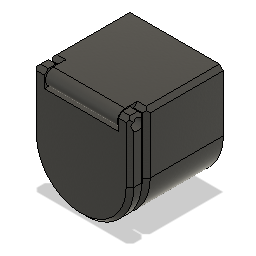
pipowerbuttoncover v2 (Autodesk Fusion 360 design; units mm, degrees)
Autodesk Fusion 360 part; units mm, degrees
sketch "Sketch1" plane through (0, 0, 0) normal (0, 0, 1) x (1, 0, 0)
  circle A0 centre (0, 0) radius 6.1
  circle A1 centre (0, 0) radius 12.5
  line L0 (-12.5, 0) -> (12.5, 0)
  line L1 (12.5, 0) -> (12.5, 12.5)
  line L2 (12.5, 12.5) -> (-12.5, 12.5)
  line L3 (-12.5, 12.5) -> (-12.5, 0)
  dimension "d1" = 12.2
  dimension "d2" = 25
  constraint coincident A0.centre A1.centre
  constraint horizontal L0
  constraint vertical L1
  constraint horizontal L2
  constraint vertical L3
  constraint midpoint A0.centre L0
  constraint coincident A1 L0.start
  constraint tangent A1 L2
  measures "d1" diameter of A0
  measures "d2" diameter of A1
extrude "Extrude1" add sketch "Sketch1" along normal blind 1 contours A0 A1 L0 | A0 A1 L0 | A1 L1 L2 | A1 L2 L3 makes body 1
sketch "Sketch2" plane through (0, 0, 1) normal (0, 0, 1) x (1, 0, 0)
  circle A0 centre (0, 0) radius 6.1
  line L0 (-12.5, 12.5) -> (-12.5, 0)
  arc A1 (-12.5, 0) -> (12.5, 0) centre (0, 0) ccw
  line L1 (12.5, 0) -> (12.5, 12.5)
  line L2 (12.5, 12.5) -> (-12.5, 12.5)
  circle A2 centre (0, 0) radius 10
  line L3 (-10, 0) -> (10, 0)
  line L4 (10, 0) -> (10, 10)
  line L5 (10, 10) -> (-10, 10)
  line L6 (-10, 10) -> (-10, 0)
  dimension "d5" = 20
  constraint concentric A0 A2
  constraint horizontal L3
  constraint vertical L4
  constraint horizontal L5
  constraint vertical L6
  constraint coincident A2 L3.start
  constraint midpoint A0.centre L3
  constraint tangent A2 L5
  measures "d5" diameter of A2
extrude "Extrude2" add sketch "Sketch2" along normal blind 19 bodies 1
extrude "Extrude3" add 3 faces at (-4.1667, 12.5, 0.3333) (8.3333, 12.5, 0.3333) (0, 12.5, 13.6667) along direction (0, 1, 0) blind 3 on bodies 1 bodies 1
sketch "Sketch3" plane through (0, 0, 20) normal (0, 0, 1) x (1, 0, 0)
  line L0 (-10, 0) -> (-10, 10)
  line L1 (-10, 10) -> (10, 10)
  line L2 (10, 10) -> (10, 0)
  arc A0 (-10, 0) -> (10, 0) centre (0, 0) ccw
  line L3 (-12.5, 15.5) -> (-12.5, 0)
  arc A1 (-12.5, 0) -> (12.5, 0) centre (0, 0) ccw
  line L4 (12.5, 0) -> (12.5, 15.5)
  line L5 (12.5, 15.5) -> (-12.5, 15.5)
extrude "Extrude4" add sketch "Sketch3" along normal blind 4 separate body contours L0 L1 L2 A0 | L3 A1 L4 L5 makes body 2
sketch "Sketch4" plane through (12.5, 0, 0) normal (1, 0, 0) x (0, 0, -1)
  line L0 (-20, 0) -> (-20, 15.5)
  line L1 (-20, 15.5) -> (-24, 15.5)
  line L2 (-24, 15.5) -> (-24, 0)
  line L3 (-24, 0) -> (-20, 0)
  line L4 (-24, 15.5) -> (-20, 15.5)
  line L5 (-20, 15.5) -> (-20, 11.5)
  line L6 (-20, 11.5) -> (-24, 11.5)
  line L7 (-24, 11.5) -> (-24, 15.5)
  circle A0 centre (-22, 13.5) radius 2
  circle A1 centre (-22, 13.5) radius 1.15
  dimension "d12" = 4
  dimension "d13" = 4
  dimension "d14" = 2.3
  constraint horizontal L4
  constraint vertical L5
  constraint horizontal L6
  constraint vertical L7
  constraint coincident L1.end L2.start
  constraint tangent L7 A0
  constraint tangent L6 A0
  constraint tangent L4 A0
  constraint concentric A0 A1
  measures "d12" distance of L1.end L0.end
  measures "d13" distance of L1.end L6.end
  measures "d14" diameter of A1
extrude "Extrude5" cut sketch "Sketch4" against normal blind 25 contours A1 bodies 2
sketch "Sketch5" plane through (12.5, 0, 0) normal (1, 0, 0) x (0, 0, -1)
  circle A0 centre (-22, 13.5) radius 1.15
  line L0 (-20, 0) -> (-20, 15.5)
  line L1 (-20, 15.5) -> (-24, 15.5)
  line L2 (-24, 15.5) -> (-24, 0)
  line L3 (-24, 0) -> (-20, 0)
  circle A1 centre (-22, 13.5) radius 1.375
  dimension "d17" = 2.75
  constraint concentric A0 A1
  measures "d17" diameter of A1
extrude "Extrude6" cut sketch "Sketch5" against normal blind 3 contours A1 bodies 2
sketch "Sketch6" plane through (-12.5, 0, 0) normal (-1, 0, 0) x (0, 0, 1)
  circle A0 centre (22, 13.5) radius 1.15
  line L0 (20, 15.5) -> (20, 0)
  line L1 (20, 0) -> (24, 0)
  line L2 (24, 0) -> (24, 15.5)
  line L3 (24, 15.5) -> (20, 15.5)
  circle A1 centre (22, 13.5) radius 1.375
  dimension "d20" = 2.75
  constraint concentric A0 A1
  measures "d20" diameter of A1
extrude "Extrude7" cut sketch "Sketch6" against normal blind 3 contours A1 bodies 2
sketch "Sketch7" plane through (0, 0, 24) normal (0, 0, 1) x (1, 0, 0)
  line L0 (12.5, 15.5) -> (-12.5, 15.5)
  line L1 (-12.5, 15.5) -> (-12.5, 0)
  arc A0 (-12.5, 0) -> (12.5, 0) centre (0, 0) ccw
  line L2 (12.5, 0) -> (12.5, 15.5)
  line L3 (-9.5, 15.5) -> (9.5, 15.5)
  line L4 (9.5, 15.5) -> (9.5, 11.5)
  line L5 (9.5, 11.5) -> (-9.5, 11.5)
  line L6 (-9.5, 11.5) -> (-9.5, 15.5)
  dimension "d23" = 4
  dimension "d24" = 3
  dimension "d25" = 3
  constraint horizontal L3
  constraint vertical L4
  constraint horizontal L5
  constraint vertical L6
  constraint coincident L0 L3.start
  measures "d23" distance of L3.start L5.end
  measures "d24" distance of L1 L6
  measures "d25" distance of L2 L4
extrude "Extrude8" cut sketch "Sketch7" against normal blind 4 contours L0 L3 L4 L5 L6 bodies 2
sketch "Sketch8" plane through (0, 0, 20) normal (0, 0, 1) x (1, 0, 0)
  line L0 (-10, 0) -> (-10, 10)
  line L1 (-10, 10) -> (10, 10)
  line L2 (10, 10) -> (10, 0)
  arc A0 (-10, 0) -> (10, 0) centre (0, 0) ccw
  line L3 (-12.5, 15.5) -> (-12.5, 0)
  arc A1 (-12.5, 0) -> (12.5, 0) centre (0, 0) ccw
  line L4 (12.5, 0) -> (12.5, 15.5)
  line L5 (12.5, 15.5) -> (-12.5, 15.5)
  line L6 (-9.5, 15.5) -> (9.5, 15.5)
  line L7 (9.5, 15.5) -> (9.5, 11.5)
  line L8 (9.5, 11.5) -> (-9.5, 11.5)
  line L9 (-9.5, 11.5) -> (-9.5, 15.5)
  point P0 (-9.5, 15.5)
  point P1 (9.5, 11.5)
  constraint horizontal L6
  constraint vertical L7
  constraint horizontal L8
  constraint vertical L9
  constraint coincident L5 P0
  constraint coincident P0 L6.start
  constraint coincident P1 L7.end
extrude "Extrude9" add sketch "Sketch8" along normal blind 4 separate body contours L5 L6 L7 L8 L9 makes body 3
sketch "Sketch9" plane through (9.5, 0, 0) normal (1, 0, 0) x (0, 0, -1)
  line L0 (-20, 11.5) -> (-20, 15.5)
  line L1 (-20, 15.5) -> (-24, 15.5)
  line L2 (-24, 15.5) -> (-24, 11.5)
  line L3 (-24, 11.5) -> (-20, 11.5)
  circle A0 centre (-22, 13.5) radius 1.125
  dimension "d30" = 2.25
  measures "d30" diameter of A0
extrude "Extrude10" cut sketch "Sketch9" against normal blind 19 contours A0 bodies 3
combine "Combine1" operation add target body 1 tool bodies 3
chamfer "Chamfer1" distance 1 angle 45 5 edges at (-12.5, 7.75, 24) (0, -12.5, 24) (12.5, 7.75, 24) (-11, 15.5, 24) (11, 15.5, 24) on bodies 2
chamfer "Chamfer2" distance 1 angle 45 5 edges at (11, 15.5, 20) (-11, 15.5, 20) (-12.5, 7.75, 20) (0, -12.5, 20) (12.5, 7.75, 20) on bodies 2
fillet "Fillet1" radius 2 2 edges at (0, 11.5, 24) (0, 15.5, 24) on bodies 1
move_face "OffsetFaces1" offset -0.25 2 faces at (-9.5, 13.5, 20.2917) (9.5, 13.5, 20.2917) on bodies 1
move_face "OffsetFaces2" offset -0.2 1 faces at (11.6667, 8.5, 20) on bodies 1
chamfer "Chamfer3" distance 1 angle 45 5 edges at (12.5, 7.75, 19.8) (-12.5, 7.75, 19.8) (0, -12.5, 19.8) (10.875, 15.5, 19.8) (-10.875, 15.5, 19.8) on bodies 1
chamfer "Chamfer4" distance 1 angle 45 4 edges at (12.5, 15.5, 9.4) (-12.5, 15.5, 9.4) (12.5, 15.5, 22) (-12.5, 15.5, 22) on bodies 1 2
chamfer "Chamfer5" distance 0.7 angle 45 1 edges at (-5.6872, 2.2059, 1) on bodies 1
